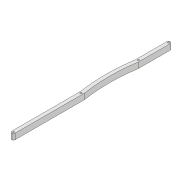
# Autodesk Inventor part: Part_7
Saved by Autodesk Inventor 2022 (Build 260153000, 153)
## iProperties
Created: 2022-05-03
Part Number: Part_7
Material: Generic
Document SubType Name: Modeling
Designer: dell
Density: 1 g/cm^3
Appearance: Default
Author: dell
Autodesk Inventor part; units mm, degrees
ref_plane "YZ Plane" through (0, 0, 0) normal (1, 0, 0) x (0, 1, 0)
ref_plane "XZ Plane" through (0, 0, 0) normal (0, 1, 0) x (-1, 0, 0)
ref_plane "XY Plane" through (0, 0, 0) normal (0, 0, 1) x (1, 0, 0)
sketch "Sketch1" plane through (0, 0, 0) normal (0, 1, 0) x (-1, 0, 0)
  line L0 (0, 0) -> (0, -270.517) construction
  line L1 (-3, 0) -> (-3, -270.517)
  line L2 (3, -270.517) -> (3, 0)
  arc A0 (3, 0) -> (-3, 0) centre (0, 0) ccw
  arc A1 (-3, -270.517) -> (3, -270.517) centre (0, -270.517) ccw
  circle A2 centre (0, 0) radius 1.5
  circle A3 centre (0, -270.517) radius 1.5
  circle A4 centre (0, -117.696) radius 1.5
  circle A5 centre (0, -217.699) radius 1.5
  arc A6 (3, -214.699) -> (3, -3) centre (-1994.197, -108.8495) ccw
  arc A7 (-3, -214.699) -> (-3, -3) centre (-2000.197, -108.8495) ccw
  circle A8 centre (3, -117.896) radius 1.5
  arc A9 (-3, -60) -> (-3, -3) centre (-98.8528, -31.5) ccw
  arc A10 (3, -60) -> (3, -3) centre (-92.8528, -31.5) ccw
  point P0 (0, -135.2585)
  point P1 (4.9983, -52.1198)
  point P2 (-1.0017, -52.1198)
  dimension "d0" = 6
  dimension "d1" = 270.517
  dimension "d2" = 3
  dimension "d3" = 3
  dimension "d10" = 3
  dimension "d11" = 117.696
  dimension "d12" = 3
  dimension "d13" = 217.699
  dimension "d22" = 2000
  dimension "d23" = 2000
  dimension "d24" = 3
  dimension "d25" = 3
  dimension "d26" = 3
  dimension "d27" = 3
  dimension "d28" = 0.2
  dimension "d29" = 100
  dimension "d30" = 100
  dimension "d31" = 60
  dimension "d33" = 60
  constraints: 12 point on circle, 11 centre point, 8 end point, 8 point on line, 4 tangent, 2 coincident, 2 horizontal alignment, 1 midpoint, 1 parallel, 1 vertical
  measures "d0" diameter of A1
  measures "d1" distance of L0.end L0.start
  measures "d2" diameter of A2
  measures "d3" diameter of A3
  measures "d10" diameter of A4
  measures "d11" distance of L0.start A4.centre
  measures "d12" diameter of A5
  measures "d13" distance of L0.start A5.centre
  measures "d22" radius of A6
  measures "d23" radius of A7
  measures "d24" horizontal distance of A5.centre A6.start
  measures "d25" horizontal distance of L0.start A6.end
  measures "d26" diameter of A8
  measures "d27" distance from line of L0 A8.centre
  measures "d28" vertical distance of A4.centre A8.centre
  measures "d29" radius of A9
  measures "d30" radius of A10
  measures "d31" vertical distance of L0.start A9.start
  measures "d33" vertical distance of L0.start A10.start
extrude "Extrusion1" add sketch "Sketch1" along normal blind 10 contours A0 L2 A8 A1 L1 A7 A4 A9 | A6 A10 L2 | A10 A6 | A4 A7 | A10 A6 L2 A8 picked at (0.3556, -117.6954)
body "Solid1"
